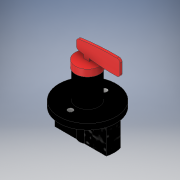
# Autodesk Inventor part: masterswitch
Saved by Autodesk Inventor 2019 (Build 230136000, 136)
## iProperties
Created: 2020-02-15
Part Number: masterswitch
Material: Generic
Document SubType Name: Modeling
Designer: brosemej
Density: 1 g/cm^3
Appearance: Default
Author: brosemej
Autodesk Inventor part; units mm, degrees
ref_plane "YZ Plane" through (0, 0, 0) normal (1, 0, 0) x (0, 1, 0)
ref_plane "XZ Plane" through (0, 0, 0) normal (0, 1, 0) x (-1, 0, 0)
ref_plane "XY Plane" through (0, 0, 0) normal (0, 0, 1) x (1, 0, 0)
sketch "Sketch1" plane through (0, 0, 0) normal (0, 1, 0) x (-1, 0, 0)
  circle A0 centre (0, 0) radius 31.75
  dimension "d0" = 63.5
  constraints: 1 centre point, 1 coincident
  measures "d0" diameter of A0
extrude "Extrusion1" add sketch "Sketch1" along normal blind 6.35
sketch "Sketch3" plane through (0, 6.35, 0) normal (0, 1, 0) x (1, 0, 0)
  circle A0 centre (0, 0) radius 12.7
  dimension "d9" = 25.4
  constraints: 1 centre point, 1 coincident
  measures "d9" diameter of A0
extrude "Extrusion3" add sketch "Sketch3" along normal blind 31.75
sketch "Sketch4" plane through (0, 38.1, 0) normal (0, 1, 0) x (1, 0, 0)
  circle A0 centre (0, 0) radius 14.9177
  constraints: 1 centre point, 1 coincident
extrude "Extrusion4" add sketch "Sketch4" along normal blind 7.62
sketch "Sketch5" plane through (0, 45.72, 0) normal (0, 1, 0) x (1, 0, 0)
  line L0 (-3.175, 1.27) -> (3.175, 1.27)
  line L1 (3.175, 1.27) -> (3.175, -1.27)
  line L2 (3.175, -1.27) -> (-3.175, -1.27)
  line L3 (-3.175, -1.27) -> (-3.175, 1.27)
  line L4 (-3.175, 1.27) -> (3.175, -1.27) construction
  line L5 (3.175, 1.27) -> (-3.175, -1.27) construction
  point P0 (0, 0)
  dimension "d14" = 6.35
  dimension "d15" = 2.54
  constraints: 12 end point, 2 midpoint, 2 parallel, 1 horizontal, 1 perpendicular
  measures "d14" distance of L1.end L2.end
  measures "d15" distance of L0.end L1.end
extrude "Extrusion5" add sketch "Sketch5" along normal blind 2.54
sketch "Sketch6" plane through (-3.175, 45.72, 1.27) normal (0, 0, 1) x (1, 0, 0)
  line L0 (-8.0078, 1.2174) -> (37.195, 1.2174)
  line L1 (40.37, 4.3924) -> (40.37, 15.4306)
  line L2 (37.195, 18.6056) -> (-8.0078, 18.6056)
  line L3 (-8.0078, 12.7012) -> (-8.0078, 7.9542)
  arc A0 (37.195, 1.2174) -> (40.37, 4.3924) centre (37.195, 4.3924) ccw
  arc A1 (40.37, 15.4306) -> (37.195, 18.6056) centre (37.195, 15.4306) ccw
  arc A2 (-5.4455, 4.8388) -> (37.195, 1.2174) centre (32.3527, 197.046) ccw
  arc A3 (37.195, 18.6056) -> (-5.2937, 15.8426) centre (33.0266, -245.3603) ccw
  arc A4 (-8.0078, 7.9542) -> (-5.4455, 4.8388) centre (-4.8328, 7.9542) ccw
  arc A5 (-5.2937, 15.8426) -> (-8.0078, 12.7012) centre (-4.8328, 12.7012) ccw
  line L4 (0, 2.54) -> (0, 3.8476)
  line L5 (6.35, 2.54) -> (0, 2.54) projected
  line L6 (6.35, 2.54) -> (6.35, 2.891)
  arc A6 (0, 3.8476) -> (6.35, 2.891) centre (32.3527, 197.046) ccw
  point P0 (3.175, -45.72)
  point P1 (-8.0078, 5.3605)
  point P2 (-8.0078, 15.43)
  dimension "d18" = 3.175
  dimension "d19" = 3.175
  constraints: 18 point on circle, 12 end point, 8 tangent, 7 centre point, 4 point on line, 3 equal radius, 2 parallel, 2 perpendicular, 1 horizontal, 1 vertical
  measures "d18" radius of A0
  measures "d19" radius of A4
extrude "Extrusion6" add sketch "Sketch6" against normal blind 2.54
sketch "Sketch7" plane through (0, 45.72, 0) normal (0, 1, 0) x (1, 0, 0)
  circle A0 centre (0, 0) radius 13.5422
  circle A1 centre (0, 0) radius 14.9177
  constraints: 2 centre point, 2 coincident
extrude "Extrusion7" cut sketch "Sketch7" against normal blind 25.4
sketch "Sketch8" plane through (0, 0, 0) normal (0, -1, 0) x (1, 0, 0)
  circle A0 centre (0, 0) radius 29.6911
  circle A1 centre (0, 0) radius 8.89
  line L0 (-4.226, 7.8213) -> (-28.6424, 7.8213)
  line L1 (4.226, 7.8213) -> (28.6424, 7.8213)
  line L2 (4.226, -7.8213) -> (28.6424, -7.8213)
  line L3 (-4.226, -7.8213) -> (-28.6424, -7.8213)
  arc A2 (-28.6424, 7.8213) -> (-28.6424, -7.8213) centre (0, 0) ccw
  arc A3 (28.6424, -7.8213) -> (28.6424, 7.8213) centre (0, 0) ccw
  dimension "d24" = 17.78
  constraints: 12 point on circle, 8 end point, 4 centre point, 4 point on line, 2 coincident, 2 concentric, 1 horizontal, 1 parallel
  measures "d24" diameter of A1
extrude "Extrusion8" add sketch "Sketch8" along normal blind 29.3624 contours A0 L2 A1 L1 | L0 A1 L3 A0 | A1
sketch "Sketch10" plane through (0, 0, 0) normal (0, -1, 0) x (1, 0, 0)
  circle A0 centre (0, 0) radius 31.75 projected
  line L0 (0, -31.75) -> (0, -19)
  line L1 (0, -19) -> (0, 31.75)
  line L2 (0, 31.75) -> (0, 19)
  circle A1 centre (0, 19) radius 2.921
  circle A2 centre (0, -19) radius 2.921
  dimension "d31" = 12.75
  dimension "d32" = 12.75
  dimension "d33" = 5.842
  constraints: 6 end point, 2 centre point, 2 coincident, 2 point on circle, 2 point on line, 1 vertical
  measures "d31" distance of L0.start L0.end
  measures "d32" distance of L1.end L2.end
  measures "d33" diameter of A1
extrude "Extrusion9" cut sketch "Sketch10" against normal blind 25.4 contours A1 L1 | L1 A1 | A2 L1 L0 | L0 L1 A2
body "Solid1"
